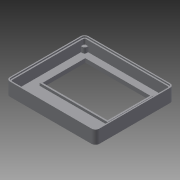
# Autodesk Inventor part: pablogilLCDCaseTop
Saved by Autodesk Inventor 2015 SP1 (Build 190203100, 203)
## iProperties
Created: 2015-04-16
Part Number: pablogilLCDCaseTop
Material: Generic
Document SubType Name: Modeling
Designer: Jack
Density: 1 g/cm^3
Appearance: Default
Author: Jack
Autodesk Inventor part; units mm, degrees
ref_plane "YZ Plane" through (0, 0, 0) normal (1, 0, 0) x (0, 1, 0)
ref_plane "XZ Plane" through (0, 0, 0) normal (0, 1, 0) x (-1, 0, 0)
ref_plane "XY Plane" through (0, 0, 0) normal (0, 0, 1) x (1, 0, 0)
sketch "Sketch1" plane through (0, 0, 0) normal (0, 0, 1) x (1, 0, 0)
  line L0 (0, 0) -> (108.6, 0)
  line L1 (108.6, 0) -> (108.6, 95.4)
  line L2 (108.6, 95.4) -> (0, 95.4)
  line L3 (0, 95.4) -> (0, 0)
  dimension "d0" = 108.6
  dimension "d1" = 95.4
  constraints: 8 end point, 2 parallel, 1 horizontal, 1 perpendicular
  measures "d0" distance of L2.end L1.end
  measures "d1" distance of L1.end L0.end
extrude "Extrusion1" add sketch "Sketch1" along normal blind 1.9
sketch "Sketch2" plane through (0, 0, 1.9) normal (0, 0, 1) x (1, 0, 0)
  line L0 (0, 0) -> (108.6, 0) projected
  line L1 (108.6, 0) -> (108.6, 95.4) projected
  line L2 (108.6, 95.4) -> (0, 95.4) projected
  line L3 (0, 95.4) -> (0, 0) projected
  line L4 (3, 92.4) -> (105.6, 92.4)
  line L5 (105.6, 92.4) -> (105.6, 3)
  line L6 (105.6, 3) -> (3, 3)
  line L7 (3, 3) -> (3, 92.4)
  dimension "d4" = 3
  constraints: 8 end point, 3 other
  measures "d4" distance between parallel lines of L2 L4
extrude "Extrusion2" add sketch "Sketch2" along normal blind 14.1
sketch "Sketch3" plane through (0, 0, 16) normal (0, 0, 1) x (1, 0, 0)
  line L0 (105.6, 92.4) -> (105.6, 3) projected
  line L1 (105.6, 3) -> (3, 3) projected
  line L2 (3, 3) -> (3, 92.4) projected
  line L3 (3, 92.4) -> (105.6, 92.4) projected
  line L4 (107.2, 94) -> (107.2, 1.4)
  line L5 (107.2, 1.4) -> (1.4, 1.4)
  line L6 (1.4, 1.4) -> (1.4, 94)
  line L7 (1.4, 94) -> (107.2, 94)
  dimension "d7" = 1.6
  constraints: 8 end point, 3 other
  measures "d7" distance between parallel lines of L3 L7
extrude "Extrusion3" cut sketch "Sketch3" against normal blind 1.5
sketch "Sketch4" plane through (0, 0, 1.9) normal (0, 0, 1) x (1, 0, 0)
  line L0 (105.6, 3) -> (105.6, 92.4) projected
  line L1 (105.6, 92.4) -> (3, 92.4) projected
  line L2 (3, 92.4) -> (3, 3) projected
  line L3 (3, 3) -> (105.6, 3) projected
  arc A0 (7.4, 4.7) -> (4.7, 7.4) centre (4.7, 4.7) ccw
  arc A1 (4.7, 88) -> (7.4, 90.7) centre (4.7, 90.7) ccw
  arc A2 (101.2, 90.7) -> (103.9, 88) centre (103.9, 90.7) ccw
  arc A3 (103.9, 7.4) -> (101.2, 4.7) centre (103.9, 4.7) ccw
  line L4 (7.4, 4.7) -> (7.4, 3)
  line L5 (3, 3) -> (105.6, 3) projected
  line L6 (4.7, 7.4) -> (3, 7.4)
  line L7 (7.4, 90.7) -> (7.4, 92.4)
  line L8 (4.7, 88) -> (3, 88)
  line L9 (101.2, 90.7) -> (101.2, 92.4)
  line L10 (103.9, 88) -> (105.6, 88)
  line L11 (103.9, 7.4) -> (105.6, 7.4)
  line L12 (101.2, 4.7) -> (101.2, 3)
  point P0 (0, 0)
  dimension "d10" = 1.7
  dimension "d11" = 1.7
  dimension "d12" = 1.7
  dimension "d13" = 1.7
  dimension "d19" = 4.4
  constraints: 16 end point, 12 point on line, 8 point on circle, 6 tangent, 5 perpendicular, 4 centre point, 4 coincident, 3 equal radius, 2 horizontal alignment, 2 vertical alignment, 1 vertical
  measures "d10" distance from line of L0 point (103.9, 90.7)
  measures "d11" distance from line of L1 point (103.9, 90.7)
  measures "d12" distance from line of L2 point (4.7, 4.7)
  measures "d13" distance from line of L3 point (4.7, 4.7)
  measures "d19" distance between parallel lines of L2 L4
extrude "Extrusion4" add sketch "Sketch4" along normal blind 5.5 contours L3 L12 A3 L11 L0 | L10 A2 L9 L1 L0 | L3 L2 L6 A0 L4 | L7 A1 L8 L2 L1
sketch "Sketch5" plane through (0, 0, 1.9) normal (0, 0, 1) x (1, 0, 0)
  line L0 (7.4, 3) -> (101.2, 3) projected
  line L1 (105.6, 7.4) -> (105.6, 88) projected
  line L2 (14.9, 29.6) -> (93.7, 29.6)
  line L3 (93.7, 29.6) -> (93.7, 81.4)
  line L4 (93.7, 81.4) -> (14.9, 81.4)
  line L5 (14.9, 81.4) -> (14.9, 29.6)
  point P0 (0, 0)
  dimension "d20" = 51.8
  dimension "d21" = 78.8
  dimension "d22" = 11.9
  dimension "d23" = 26.6
  constraints: 8 end point, 2 parallel, 1 horizontal, 1 perpendicular
  measures "d20" distance of L4.end L2.start
  measures "d21" distance of L2.start L2.end
  measures "d22" distance between parallel lines of L1 L3
  measures "d23" distance between parallel lines of L0 L2
extrude "Extrusion5" cut sketch "Sketch5" against normal up to next
sketch "Sketch6" plane through (0, 0, 1.9) normal (0, 0, 1) x (1, 0, 0)
  line L0 (93.7, 81.4) -> (93.7, 29.6) projected
  line L1 (93.7, 29.6) -> (14.9, 29.6) projected
  line L2 (14.9, 29.6) -> (14.9, 81.4) projected
  line L3 (14.9, 81.4) -> (93.7, 81.4) projected
  line L4 (95.6, 83.3) -> (95.6, 27.7)
  line L5 (95.6, 27.7) -> (13, 27.7)
  line L6 (13, 27.7) -> (13, 83.3)
  line L7 (13, 83.3) -> (95.6, 83.3)
  point P0 (0, 0)
  dimension "d26" = 1.9
  constraints: 8 end point, 3 other
  measures "d26" distance between parallel lines of L3 L7
extrude "Extrusion6" add sketch "Sketch6" along normal blind 3
fillet "Fillet1" radius 4.7 4 edges at (0, 95.4, 8) (108.6, 95.4, 8) (108.6, 0, 8) (0, 0, 8)
fillet "Fillet2" radius 3.3 4 edges at (107.2, 1.4, 15.25) (1.4, 1.4, 15.25) (1.4, 94, 15.25) (107.2, 94, 15.25)
fillet "Fillet3" radius 1.7 4 edges at (3, 3, 10.95) (3, 92.4, 10.95) (105.6, 92.4, 10.95) (105.6, 3, 10.95)
body "Solid1"
